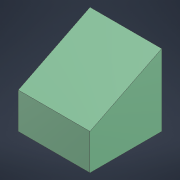
# Autodesk Inventor part: 110033226_ipt_14_草地三
Saved by Autodesk Inventor 2022 (Build 260153000, 153)
## iProperties
Created: 2022-06-22
Part Number: 110033226_ipt_14_草地三
Material: 一般
Document SubType Name: Modeling
Designer: User
Density: 1 g/cm^3
Appearance: 預設
Author: User
Autodesk Inventor part; units mm, degrees
ref_plane "YZ Plane" through (0, 0, 0) normal (1, 0, 0) x (0, 1, 0)
ref_plane "XZ Plane" through (0, 0, 0) normal (0, 1, 0) x (-1, 0, 0)
ref_plane "XY Plane" through (0, 0, 0) normal (0, 0, 1) x (1, 0, 0)
sketch "草圖1" plane through (0, 0, 0) normal (0, 1, 0) x (-1, 0, 0)
  line L0 (2.5, 2.5) -> (-2.5, 2.5)
  line L1 (-2.5, 2.5) -> (-2.5, -2.5)
  line L2 (-2.5, -2.5) -> (2.5, -2.5)
  line L3 (2.5, -2.5) -> (2.5, 2.5)
  circle A0 centre (0, 0) radius 1.7
  point P0 (0, -2.5)
  point P1 (2.5, 0)
  dimension "d0" = 5
  dimension "d1" = 5
  dimension "d2" = 3.4
  constraints: 8 end point, 2 midpoint, 2 parallel, 1 centre point, 1 coincident, 1 horizontal, 1 horizontal alignment, 1 perpendicular, 1 vertical alignment
  measures "d0" distance of L2.end L1.end
  measures "d1" distance of L1.end L0.end
  measures "d2" diameter of A0
sketch "草圖2" plane through (0, 0, 0) normal (1, 0, 0) x (0, 1, 0)
  line L0 (0, -2.5) -> (0, 2.5) projected
  line L1 (5, -2.5) -> (0, -2.5)
  line L2 (0, 0) -> (1.5, 0)
  line L3 (0, 2.5) -> (2.5, 2.5)
  line L4 (2.5, 2.5) -> (5, -2.5)
  point P0 (0, 2.5)
  dimension "d3" = 1.5
  dimension "d7" = 2.5
  dimension "d8" = 5
  constraints: 8 end point, 2 horizontal, 1 perpendicular
  measures "d3" distance of L2.start L2.end
  measures "d7" distance of L3.start L3.end
  measures "d8" distance of L1.start L0.start
extrude "擠出1" add sketch "草圖2" along normal mid plane 5
extrude "擠出2" cut sketch "草圖1" along normal blind 1.5 contours A0
